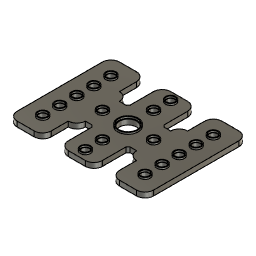
Robotic_arm_2 (Autodesk Fusion 360 design; units mm, degrees)
Autodesk Fusion 360 part; units mm, degrees
note: some values were not read from the file. Set by a fixed rule: which sketch regions a step uses.
sketch "Esquisse1" plane through (0, 0, 0) normal (0, 0, 1) x (1, 0, 0)
  line L0 (40, -10) -> (-40, -10)
  line L1 (-40, -10) -> (-40, 10)
  line L2 (-40, 10) -> (40, 10)
  line L3 (40, 10) -> (40, -10)
  line L4 (40, -10) -> (-40, 10) construction
  line L5 (-40, -10) -> (40, 10) construction
  line L6 (-40, -10) -> (-20, -10)
  line L7 (-20, -10) -> (-20, 25)
  line L8 (-25, 30) -> (-35, 30)
  line L9 (-40, 25) -> (-40, -10)
  line L10 (-40, 10) -> (-20, 10)
  line L11 (-20, 10) -> (-20, -25)
  line L12 (-25, -30) -> (-35, -30)
  line L13 (-40, -25) -> (-40, 10)
  line L14 (40, -10) -> (20, -10)
  line L15 (20, -10) -> (20, 25)
  line L16 (25, 30) -> (35, 30)
  line L17 (40, 25) -> (40, -10)
  line L18 (40, 10) -> (20, 10)
  line L19 (20, 10) -> (20, -25)
  line L20 (25, -30) -> (35, -30)
  line L21 (40, -25) -> (40, 10)
  circle A0 centre (-30, 20) radius 2.25
  circle A1 centre (30, 20) radius 2.25
  circle A2 centre (-30, -20) radius 2.25
  circle A3 centre (30, -20) radius 2.25
  circle A4 centre (0, 0) radius 5
  circle A5 centre (-20, 10) radius 5
  circle A6 centre (20, 10) radius 5
  circle A7 centre (-20, -10) radius 5
  circle A8 centre (20, -10) radius 5
  circle A9 centre (-30, 0) radius 2.25
  circle A10 centre (30, 0) radius 2.25
  circle A11 centre (-30, 10) radius 2.25
  circle A12 centre (30, 10) radius 2.25
  circle A13 centre (-30, -10) radius 2.25
  circle A14 centre (30, -10) radius 2.25
  arc A15 (-25, -30) -> (-20, -25) centre (-25, -25) ccw
  arc A16 (-40, -25) -> (-35, -30) centre (-35, -25) ccw
  arc A17 (-35, 30) -> (-40, 25) centre (-35, 25) ccw
  arc A18 (-20, 25) -> (-25, 30) centre (-25, 25) ccw
  arc A19 (25, 30) -> (20, 25) centre (25, 25) ccw
  arc A20 (40, 25) -> (35, 30) centre (35, 25) ccw
  arc A21 (35, -30) -> (40, -25) centre (35, -25) ccw
  circle A22 centre (0, 0) radius 15
  arc A23 (20, -25) -> (25, -30) centre (25, -25) ccw
  line L22 (5, 30) -> (-5, 30)
  line L23 (-10, 25) -> (-10, -25)
  line L24 (-5, -30) -> (5, -30)
  line L25 (10, -25) -> (10, 25)
  circle A24 centre (0, 25) radius 2.25
  circle A25 centre (0, -25) radius 2.25
  circle A26 centre (0, -15) radius 2.25
  circle A27 centre (0, 15) radius 2.25
  arc A28 (-5, 30) -> (-10, 25) centre (-5, 25) ccw
  arc A29 (10, 25) -> (5, 30) centre (5, 25) ccw
  arc A30 (-10, -25) -> (-5, -30) centre (-5, -25) ccw
  arc A31 (5, -30) -> (10, -25) centre (5, -25) ccw
  circle A32 centre (-15, 0) radius 2.25
  circle A33 centre (15, 0) radius 2.25
  point P0 (-40, 30)
  point P1 (-40, -30)
  point P2 (40, 30)
  point P3 (40, -30)
  point P4 (-10, 30)
  point P5 (-10, -30)
  point P6 (10, -30)
  dimension "d1" = 80
  dimension "d2" = 20
  dimension "d3" = 20
  dimension "d4" = 40
  dimension "d5" = 20
  dimension "d6" = 40
  dimension "d7" = 20
  dimension "d8" = 40
  dimension "d9" = 20
  dimension "d10" = 40
  dimension "d11" = 4.5
  dimension "d12" = 4.5
  dimension "d13" = 4.5
  dimension "d14" = 4.5
  dimension "d15" = 10
  dimension "d16" = 10
  dimension "d17" = 10
  dimension "d18" = 10
  dimension "d19" = 10
  dimension "d20" = 4.5
  dimension "d21" = 4.5
  dimension "d22" = 4.5
  dimension "d23" = 4.5
  dimension "d24" = 4.5
  dimension "d25" = 4.5
  dimension "d28" = 5
  dimension "d29" = 30
  dimension "d30" = 5
  dimension "d31" = 20
  dimension "d32" = 60
  dimension "d33" = 4.5
  dimension "d34" = 4.5
  dimension "d35" = 4.5
  dimension "d36" = 4.5
  dimension "d37" = 5
  dimension "d38" = 5
  dimension "d39" = 5
  dimension "d40" = 5
  dimension "d41" = 4.5
  dimension "d42" = 4.5
  constraint horizontal L0
  constraint perpendicular L0 L1
  constraint parallel L0 L2
  constraint parallel L1 L3
  constraint coincident L4 A4.centre
  constraint coincident L5 A4.centre
  constraint coincident A4.centre A22.centre
  constraint horizontal L6
  constraint vertical L7
  constraint horizontal L8
  constraint vertical L9
  constraint horizontal L10
  constraint vertical L11
  constraint horizontal L12
  constraint vertical L13
  constraint horizontal L14
  constraint vertical L15
  constraint horizontal L16
  constraint vertical L17
  constraint horizontal L18
  constraint vertical L19
  constraint horizontal L20
  constraint vertical L21
  constraint coincident L10.end L11.start
  constraint coincident L18.end L19.start
  constraint coincident L6.end L7.start
  constraint coincident L14.end L15.start
  constraint midpoint L10 A11.centre
  constraint midpoint L18 A12.centre
  constraint midpoint L6 A13.centre
  constraint midpoint L14 A14.centre
  constraint tangent L11 A15
  constraint tangent L12 A15
  constraint coincident P1 L12
  constraint coincident P1 L13
  constraint tangent L12 A16
  constraint tangent L13 A16
  constraint equal A15 A16
  constraint coincident P0 L8
  constraint coincident P0 L9
  constraint tangent L8 A17
  constraint tangent L9 A17
  constraint equal A15 A17
  constraint tangent L7 A18
  constraint tangent L8 A18
  constraint equal A15 A18
  constraint tangent L15 A19
  constraint tangent L16 A19
  constraint equal A15 A19
  constraint coincident P2 L16
  constraint coincident P2 L17
  constraint tangent L16 A20
  constraint tangent L17 A20
  constraint equal A15 A20
  constraint coincident P3 L20
  constraint coincident P3 L21
  constraint tangent L20 A21
  constraint tangent L21 A21
  constraint equal A15 A21
  constraint tangent L19 A23
  constraint tangent L20 A23
  constraint horizontal L22
  constraint perpendicular L22 L23
  constraint parallel L22 L24
  constraint parallel L23 L25
  constraint coincident A22 A26.centre
  constraint coincident A22 A27.centre
  constraint coincident P4 L22
  constraint coincident P4 L23
  constraint tangent L22 A28
  constraint tangent L23 A28
  constraint tangent L22 A29
  constraint tangent L25 A29
  constraint coincident P5 L23
  constraint coincident P5 L24
  constraint tangent L23 A30
  constraint tangent L24 A30
  constraint coincident P6 L24
  constraint coincident P6 L25
  constraint tangent L24 A31
  constraint tangent L25 A31
  constraint coincident A22 A32.centre
  constraint coincident A22 A33.centre
  measures "d1" distance of L1.end L2.end
  measures "d2" distance of L0.end L1.end
  measures "d3" distance of L0.end L6.end
  measures "d4" distance of L0.end P0
  measures "d5" distance of L1.end L10.end
  measures "d6" distance of L1.end P1
  measures "d7" distance of L0.start L14.end
  measures "d8" distance of L0.start P2
  measures "d9" distance of L2.end L18.end
  measures "d10" distance of L2.end P3
  measures "d11" diameter of A0
  measures "d12" diameter of A1
  measures "d13" diameter of A2
  measures "d14" diameter of A3
  measures "d15" diameter of A4
  measures "d16" diameter of A5
  measures "d17" diameter of A6
  measures "d18" diameter of A7
  measures "d19" diameter of A8
  measures "d20" diameter of A9
  measures "d21" diameter of A10
  measures "d22" diameter of A11
  measures "d23" diameter of A12
  measures "d24" diameter of A13
  measures "d25" diameter of A14
  measures "d28" radius of A15
  measures "d29" diameter of A22
  measures "d30" radius of A23
  measures "d31" distance of P5 P6
  measures "d32" distance of P4 P5
  measures "d33" diameter of A24
  measures "d34" diameter of A25
  measures "d35" diameter of A26
  measures "d36" diameter of A27
  measures "d37" radius of A28
  measures "d38" radius of A29
  measures "d39" radius of A30
  measures "d40" radius of A31
  measures "d41" diameter of A32 L11
  measures "d42" diameter of A33 L11
extrude "Extrusion1" add sketch "Esquisse1" against normal blind 3 contours L0 L14 L19 L20 L21 A8 A14 A21 A23 | L0 L2 L3 L14 L15 L17 L18 L19 L21 A6 A8 A12 A14 | L2 L15 L16 L17 L18 A6 A12 A19 A20 | L0 L14 L19 A8 | L0 L14 L15 L19 A8 | L0 L19 A8 | L0 L15 L19 A8 | L0 L2 L15 L19 A6 A8 A22 A33 | L2 L15 L18 L19 A6 | L2 L15 L18 A6 | L2 L15 L19 A6 | L2 L15 A6 | L0 A22 L25 | L0 L2 A22 L25 A33 | L0 A22 L23 L25 A26 | L0 L2 L23 L25 | A22 L23 L24 L25 A26 A30 A31 | L2 A22 L25 | L0 A22 L23 | L0 L2 A22 L23 A32 | L2 A22 L23 L25 A27 | A22 L22 L23 L25 A27 A28 A29 | L0 L2 L7 L11 A5 A7 A22 A32 | L2 A22 L23 | L0 L11 A7 | L0 L7 L11 A7 | L0 L6 L11 A7 | L0 L6 L7 L11 A7 | L0 L1 L2 L6 L7 L9 L10 L11 L13 A5 A7 A11 A13 | L0 L6 L11 L12 L13 A7 A13 A15 A16 | L2 L7 L11 A5 | L2 L7 A5 | L2 L7 L10 L11 A5 | L2 L7 L10 A5 | L2 L7 L8 L9 L10 A5 A11 A17 A18
sketch "Esquisse2" plane through (0, 0, 0) normal (0, 0, 1) x (1, 0, 0)
  circle A0 centre (30, 10) radius 2.25
  circle A1 centre (0, -15) radius 2.25
  circle A2 centre (-30, 20) radius 2.25
  circle A3 centre (30, 20) radius 2.25
  circle A4 centre (0, -25) radius 2.25
  circle A5 centre (0, 25) radius 2.25
  circle A6 centre (-30, 10) radius 2.25
  circle A7 centre (30, 0) radius 2.25
  circle A8 centre (-30, 0) radius 2.25
  circle A9 centre (0, 0) radius 5
  circle A10 centre (30, -20) radius 2.25
  circle A11 centre (-30, -20) radius 2.25
  circle A12 centre (-30, -10) radius 2.25
  circle A13 centre (0, 15) radius 2.25
  circle A14 centre (-15, 0) radius 2.25
  circle A15 centre (15, 0) radius 2.25
  circle A16 centre (30, -10) radius 2.25
  arc A17 (-11.1803, -10) -> (-10, -11.1803) centre (0, 0) ccw
  line L0 (-10, -11.1803) -> (-10, -25)
  arc A18 (-10, -25) -> (-5, -30) centre (-5, -25) ccw
  line L1 (-5, -30) -> (5, -30)
  arc A19 (5, -30) -> (10, -25) centre (5, -25) ccw
  line L2 (10, -25) -> (10, -11.1803)
  arc A20 (10, -11.1803) -> (11.1803, -10) centre (0, 0) ccw
  line L3 (11.1803, -10) -> (15, -10)
  arc A21 (15, -10) -> (20, -15) centre (20, -10) ccw
  line L4 (20, -15) -> (20, -25)
  arc A22 (20, -25) -> (25, -30) centre (25, -25) ccw
  line L5 (25, -30) -> (35, -30)
  arc A23 (35, -30) -> (40, -25) centre (35, -25) ccw
  line L6 (40, -25) -> (40, 25)
  arc A24 (40, 25) -> (35, 30) centre (35, 25) ccw
  line L7 (35, 30) -> (25, 30)
  arc A25 (25, 30) -> (20, 25) centre (25, 25) ccw
  line L8 (20, 25) -> (20, 15)
  arc A26 (20, 15) -> (15, 10) centre (20, 10) ccw
  line L9 (15, 10) -> (11.1803, 10)
  arc A27 (11.1803, 10) -> (10, 11.1803) centre (0, 0) ccw
  line L10 (10, 11.1803) -> (10, 25)
  arc A28 (10, 25) -> (5, 30) centre (5, 25) ccw
  line L11 (5, 30) -> (-5, 30)
  arc A29 (-5, 30) -> (-10, 25) centre (-5, 25) ccw
  line L12 (-10, 25) -> (-10, 11.1803)
  arc A30 (-10, 11.1803) -> (-11.1803, 10) centre (0, 0) ccw
  line L13 (-11.1803, 10) -> (-15, 10)
  arc A31 (-15, 10) -> (-20, 15) centre (-20, 10) ccw
  line L14 (-20, 15) -> (-20, 25)
  arc A32 (-20, 25) -> (-25, 30) centre (-25, 25) ccw
  line L15 (-25, 30) -> (-35, 30)
  arc A33 (-35, 30) -> (-40, 25) centre (-35, 25) ccw
  line L16 (-40, 25) -> (-40, -25)
  arc A34 (-40, -25) -> (-35, -30) centre (-35, -25) ccw
  line L17 (-35, -30) -> (-25, -30)
  arc A35 (-25, -30) -> (-20, -25) centre (-25, -25) ccw
  line L18 (-20, -25) -> (-20, -15)
  arc A36 (-20, -15) -> (-15, -10) centre (-20, -10) ccw
  line L19 (-15, -10) -> (-11.1803, -10)
  circle A37 centre (0, 25) radius 2.5
  circle A38 centre (0, 25) radius 3
  circle A39 centre (0, 15) radius 2.5
  circle A40 centre (-15, 0) radius 2.5
  circle A41 centre (-30, 10) radius 3
  circle A42 centre (-30, 20) radius 2.5
  circle A43 centre (-30, 0) radius 2.5
  circle A44 centre (-30, -10) radius 2.5
  circle A45 centre (-30, -20) radius 2.5
  circle A46 centre (0, -15) radius 2.5
  circle A47 centre (0, -25) radius 2.5
  circle A48 centre (15, 0) radius 2.5
  circle A49 centre (30, 10) radius 2.5
  circle A50 centre (30, 20) radius 2.5
  circle A51 centre (30, 0) radius 2.5
  circle A52 centre (30, -10) radius 2.5
  circle A53 centre (30, -20) radius 2.5
  circle A54 centre (0, 15) radius 3
  circle A55 centre (-15, 0) radius 3
  circle A56 centre (-30, 0) radius 3
  circle A57 centre (-30, 10) radius 2.5
  circle A58 centre (-30, 20) radius 3
  circle A59 centre (-30, -10) radius 3
  circle A60 centre (-30, -20) radius 3
  circle A61 centre (0, -15) radius 3
  circle A62 centre (0, -25) radius 3
  circle A63 centre (15, 0) radius 3
  circle A64 centre (30, 20) radius 3
  circle A65 centre (30, 10) radius 3
  circle A66 centre (30, 0) radius 3
  circle A67 centre (30, -10) radius 3
  circle A68 centre (30, -20) radius 3
  circle A69 centre (0, 0) radius 5.5
  circle A70 centre (0, 0) radius 6
  dimension "d43" = 5
  dimension "d44" = 6
  dimension "d45" = 5
  dimension "d46" = 5
  dimension "d47" = 6
  dimension "d48" = 5
  dimension "d49" = 5
  dimension "d50" = 5
  dimension "d51" = 5
  dimension "d52" = 5
  dimension "d53" = 5
  dimension "d54" = 5
  dimension "d55" = 5
  dimension "d56" = 5
  dimension "d57" = 5
  dimension "d58" = 5
  dimension "d59" = 5
  dimension "d60" = 6
  dimension "d61" = 6
  dimension "d62" = 6
  dimension "d63" = 5
  dimension "d64" = 6
  dimension "d65" = 6
  dimension "d66" = 6
  dimension "d67" = 6
  dimension "d68" = 6
  dimension "d69" = 6
  dimension "d70" = 6
  dimension "d71" = 6
  dimension "d72" = 6
  dimension "d73" = 6
  dimension "d74" = 6
  dimension "d75" = 11
  dimension "d76" = 12
  constraint concentric A5 A37
  constraint concentric A37 A38
  constraint concentric A13 A39
  constraint concentric A14 A40
  constraint concentric A6 A41
  constraint concentric A2 A42
  constraint concentric A8 A43
  constraint concentric A12 A44
  constraint concentric A11 A45
  constraint concentric A1 A46
  constraint concentric A4 A47
  constraint concentric A15 A48
  constraint concentric A0 A49
  constraint concentric A3 A50
  constraint concentric A7 A51
  constraint concentric A16 A52
  constraint concentric A10 A53
  constraint concentric A13 A54
  constraint concentric A40 A55
  constraint concentric A43 A56
  constraint concentric A41 A57
  constraint concentric A2 A58
  constraint concentric A44 A59
  constraint concentric A45 A60
  constraint concentric A46 A61
  constraint concentric A47 A62
  constraint concentric A48 A63
  constraint concentric A50 A64
  constraint concentric A0 A65
  constraint concentric A51 A66
  constraint concentric A52 A67
  constraint concentric A10 A68
  constraint concentric A9 A69
  constraint concentric A9 A70
  measures "d40" radius of L13.end
  measures "d43" diameter of A37
  measures "d44" diameter of A38
  measures "d45" diameter of A39
  measures "d46" diameter of A40
  measures "d47" diameter of A41
  measures "d48" diameter of A42
  measures "d49" diameter of A43
  measures "d50" diameter of A44
  measures "d51" diameter of A45
  measures "d52" diameter of A46
  measures "d53" diameter of A47
  measures "d54" diameter of A48
  measures "d55" diameter of A49
  measures "d56" diameter of A50
  measures "d57" diameter of A51
  measures "d58" diameter of A52
  measures "d59" diameter of A53
  measures "d60" diameter of A54
  measures "d61" diameter of A55
  measures "d62" diameter of A56
  measures "d63" diameter of A57
  measures "d64" diameter of A58
  measures "d65" diameter of A59
  measures "d66" diameter of A60
  measures "d67" diameter of A61
  measures "d68" diameter of A62
  measures "d69" diameter of A63
  measures "d70" diameter of A64
  measures "d71" diameter of A65
  measures "d72" diameter of A66
  measures "d73" diameter of A67
  measures "d74" diameter of A68
  measures "d75" diameter of A69
  measures "d76" diameter of A70
extrude "Extrusion2" add sketch "Esquisse2" along normal blind 1 contours A38 | A41 | A54 | A55 | A56 | A58 | A59 | A60 | A61 | A62 | A63 | A64 | A65 | A66 | A67 | A68 | A70
